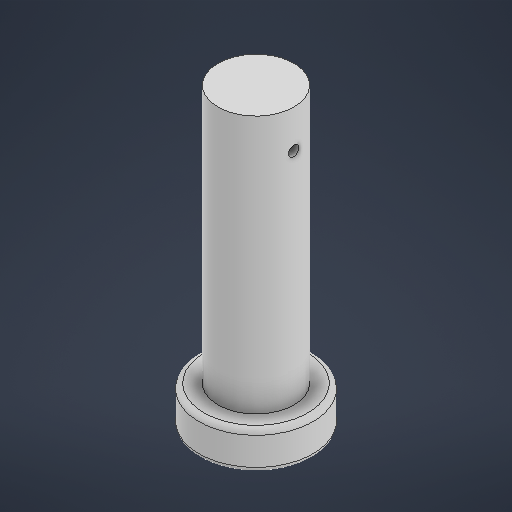
# Autodesk Inventor part: pin
Saved by Autodesk Inventor 2026.3 (Build 303398000, 398)
## iProperties
Created: 2026-07-15
Part Number: pin
Material: Generic
Document SubType Name: Modeling
Designer: User
Density: 1 g/cm^3
Appearance: Default
Author: User
Autodesk Inventor part; units mm, degrees
ref_plane "YZ Plane" through (0, 0, 0) normal (1, 0, 0) x (0, 1, 0)
ref_plane "XZ Plane" through (0, 0, 0) normal (0, 1, 0) x (-1, 0, 0)
ref_plane "XY Plane" through (0, 0, 0) normal (0, 0, 1) x (1, 0, 0)
sketch "Sketch1" plane through (0, 0, 0) normal (0, 1, 0) x (-1, 0, 0)
  circle A0 centre (0, 0) radius 22.5
  dimension "d0" = 45
  constraints: 1 centre point, 1 coincident
  measures "d0" diameter of A0
extrude "Extrusion1" add sketch "Sketch1" along normal blind 15
sketch "Sketch2" plane through (0, 15, 0) normal (0, 1, 0) x (1, 0, 0)
  circle A0 centre (0, 0) radius 15
  dimension "d3" = 30
  constraints: 1 centre point, 1 coincident
  measures "d3" diameter of A0
extrude "Extrusion2" add sketch "Sketch2" along normal blind 102
sketch "Sketch3" plane through (0, 0, 0) normal (0, 0, 1) x (1, 0, 0)
  line L0 (-15, 15) -> (-15, 117) projected
  line L1 (-15, 102) -> (15, 102)
  line L2 (15, 15) -> (15, 117) projected
  line L3 (15, 117) -> (-15, 117) projected
  line L4 (-15, 102) -> (-15, 105)
  line L5 (15, 102) -> (15, 104)
  line L6 (15, 104) -> (-15, 105)
  point P0 (0, 0)
  dimension "d6" = 15
  dimension "d7" = 3
  dimension "d8" = 2
  constraints: 8 end point, 4 point on line, 1 horizontal
  measures "d6" distance between parallel lines of L3 L1
  measures "d7" distance of L1.start L4.end
  measures "d8" distance of L1.end L5.end
revolve "Revolution1" cut sketch "Sketch3" angle 360 about axis through (-15, 102, 0) along (1, 0, 0) contours L0 L6 L2 L1
fillet "Fillet1" radius 2 2 edges at (22.5, 15, 0) (22.5, 0, 0)
body "Solid1"
